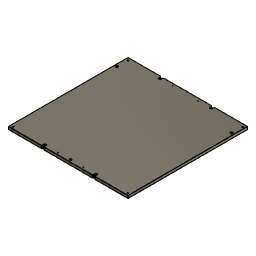
Voron_Universal_350x350_BuildPlate (Autodesk Fusion 360 design; units mm, degrees)
Autodesk Fusion 360 part; units mm, degrees
note: some values were not read from the file. Chosen so that the rebuilt part matches the saved one: how an offset face is resized; which pieces of a blend or face edit are solid.
sketch "Sketch1" plane through (0, 0, 0) normal (0, 1, 0) x (1, 0, 0)
  line L0 (0, 0) -> (351.6, 0)
  line L1 (351.6, 0) -> (351.6, 351.6)
  line L2 (351.6, 351.6) -> (0, 351.6)
  line L3 (0, 351.6) -> (0, 0)
  line L4 (175.8, 0) -> (100.8, 0)
  line L5 (100.8, 0) -> (100.8, 7)
  line L6 (100.8, 7) -> (175.8, 7) construction
  line L7 (175.8, 7) -> (175.8, 0) construction
  line L8 (351.6, 175.8) -> (300, 175.8) construction
  circle A0 centre (100.8, 7) radius 1.7
  circle A1 centre (250.8, 7) radius 1.7
  circle A2 centre (250.8, 344.6) radius 1.7
  circle A3 centre (100.8, 344.6) radius 1.7
  line L9 (0, 0) -> (7, 0)
  line L10 (7, 0) -> (7, 7) construction
  line L11 (7, 7) -> (0, 7) construction
  line L12 (0, 7) -> (0, 0)
  line L13 (351.6, 0) -> (344.6, 0)
  line L14 (344.6, 0) -> (344.6, 7) construction
  line L15 (344.6, 7) -> (351.6, 7) construction
  line L16 (351.6, 7) -> (351.6, 0)
  circle A4 centre (344.6, 7) radius 2.1
  circle A5 centre (7, 7) radius 2.1
  point P0 (250.8, 7)
  dimension "d1" = 351.6
  dimension "d2" = 351.6
  dimension "d3" = 75
  dimension "d4" = 7
  dimension "d5" = 3.4
  dimension "d6" = 7
  dimension "d7" = 7
  dimension "d8" = 7
  dimension "d9" = 7
  dimension "d10" = 4.2
  dimension "d11" = 4.2
  constraint horizontal L0
  constraint vertical L1
  constraint horizontal L2
  constraint vertical L3
  constraint coincident L0.start L3.end
  constraint horizontal L4
  constraint vertical L5
  constraint horizontal L6
  constraint vertical L7
  constraint midpoint L0 L4.start
  constraint midpoint L1 L8.start
  constraint perpendicular L1 L8
  constraint coincident L5.end L6.start
  constraint symmetric L7 L5.end P0
  constraint symmetric L7 A0 A1
  constraint symmetric L8 A0 A3
  constraint symmetric L8 A1 A2
  constraint horizontal L9
  constraint vertical L10
  constraint horizontal L11
  constraint vertical L12
  constraint horizontal L13
  constraint vertical L14
  constraint horizontal L15
  constraint vertical L16
  constraint coincident L14.end L15.start
  constraint coincident L10.end L11.start
  measures "d1" distance of L0.start L0.end
  measures "d2" distance of L0.start L2.end
  measures "d3" distance of L4.start L4.end
  measures "d4" distance of L4.start L6.end
  measures "d5" diameter of A0
  measures "d6" distance of L0.start L9.end
  measures "d7" distance of L0.start L11.end
  measures "d8" distance of L0.end L13.end
  measures "d9" distance of L0.end L15.end
  measures "d10" diameter of A4
  measures "d11" diameter of A5
extrude "Extrude1" add sketch "Sketch1" along normal blind 8 makes body 1
sketch "Sketch2" plane through (0, 8, 0) normal (0, 1, 0) x (-1, 0, 0)
  circle A0 centre (-250.8, -7) radius 1.7
  circle A1 centre (-250.8, -344.6) radius 1.7
  circle A2 centre (-100.8, -7) radius 1.7
  circle A3 centre (-344.6, -7) radius 2.1
  circle A4 centre (-7, -7) radius 2.1
  circle A5 centre (-100.8, -344.6) radius 1.7
  line L0 (-351.6, -351.6) -> (0, -351.6)
  line L1 (0, -351.6) -> (0, 0)
  line L2 (0, 0) -> (-351.6, 0)
  line L3 (-351.6, 0) -> (-351.6, -351.6)
  circle A6 centre (-100.8, -344.6) radius 3.25
  circle A7 centre (-250.8, -344.6) radius 3.25
  circle A8 centre (-100.8, -7) radius 3.25
  circle A9 centre (-250.8, -7) radius 3.25
  dimension "d14" = 6.5
  dimension "d15" = 6.5
  dimension "d16" = 6.5
  dimension "d17" = 6.5
  constraint concentric A5 A6
  constraint concentric A1 A7
  constraint concentric A2 A8
  constraint concentric A0 A9
  measures "d14" diameter of A6
  measures "d15" diameter of A7
  measures "d16" diameter of A8
  measures "d17" diameter of A9
extrude "Extrude2" cut sketch "Sketch2" against normal blind 3.5 contours A6 | A7 | A8 | A9 bodies 1
delete_face "DeleteFace1" 1 faces at (345.4637, 5.3333, -8.9142) on bodies 1
delete_face "DeleteFace2" 1 faces at (9.0974, 5.3333, -6.8953) on bodies 1
extrude "Extrude3" cut sketch "Sketch1" along normal blind 6 contours A4 | A5 bodies 1
thread "Thread1" "ISO Metric profile 5.0 M5x0.8 6H" major diameter 5.12 minor diameter 4.234 pitch 0.8 angle 60 resizes the face on face at (9.0974, 4, -6.8953) on face at (345.4637, 4, -8.9142) on bodies 1
copy_body "Body->Comp1" bodies 1 removing the originals makes body 2 in component "Component"
chamfer "Chamfer1" distance 0.2 angle 45 8 edges at (0, 0, -175.8) (175.8, 0, 0) (0, 8, -175.8) (175.8, 8, -351.6) (175.8, 0, -351.6) (351.6, 0, -175.8) (351.6, 8, -175.8) (175.8, 8, 0) on bodies 2 in component "Component"
fillet "Fillet1" radius 0.2 4 edges at (351.6, 4, 0) (0, 4, 0) (351.6, 4, -351.6) (0, 4, -351.6) on bodies 2 in component "Component"
delete_face "DeleteFace1'" 8 faces at (117.2667, 7.9333, -0.1333) (351.4667, 7.9333, -117.2667) (117.2667, 7.8667, -351.5333) (0.0667, 7.8667, -117.2667) (0.1333, 0.0667, -234.3333) (117.2667, 0.1333, -351.5333) (234.3333, 0.1333, -0.0667) (351.4667, 0.0667, -117.2667) on bodies 2 in component "Component"
sketch "Sketch3" plane through (0, 8, 0) normal (0, 1, 0) x (-1, 0, 0)
  line L0 (0, -351.4) -> (0, -0.2)
  arc A0 (0, -0.2) -> (-0.2, 0) centre (-0.2, -0.2) ccw
  line L1 (-0.2, 0) -> (-351.4, 0)
  arc A1 (-351.4, 0) -> (-351.6, -0.2) centre (-351.4, -0.2) ccw
  line L2 (-351.6, -0.2) -> (-351.6, -351.4)
  arc A2 (-351.6, -351.4) -> (-351.4, -351.6) centre (-351.4, -351.4) ccw
  line L3 (-351.4, -351.6) -> (-0.2, -351.6)
  arc A3 (-0.2, -351.6) -> (0, -351.4) centre (-0.2, -351.4) ccw
  circle A4 centre (-250.8, -344.6) radius 3.25
  circle A5 centre (-250.8, -7) radius 3.25
  circle A6 centre (-100.8, -344.6) radius 3.25
  circle A7 centre (-100.8, -7) radius 3.25
  line L4 (-250.8, -7) -> (-254.05, -7) construction
  line L5 (-250.8, -7) -> (-247.55, -7) construction
  line L6 (-254.05, -7) -> (-254.05, 0)
  line L7 (-247.55, -7) -> (-247.55, 0)
  constraint coincident A5.centre L4.start
  constraint coincident A5 L4.end
  constraint horizontal L4
  constraint coincident A5 L5.end
  constraint parallel L4 L5
  constraint coincident L1 L6.end
  constraint tangent A5 L6
  constraint coincident L1 L7.end
  constraint tangent A5 L7
extrude "Extrude1'" cut sketch "Sketch3" against normal blind 3.5 contours L1 A5 L6 L7 bodies 2 in component "Component"
sketch "Sketch4" plane through (0, 4.5, 0) normal (0, 1, 0) x (-1, 0, 0)
  circle A0 centre (-250.8, -7) radius 1.7
  arc A1 (-254.05, -7) -> (-247.55, -7) centre (-250.8, -7) ccw
  line L0 (-247.55, -7) -> (-247.55, 0)
  line L1 (-247.55, 0) -> (-254.05, 0)
  line L2 (-254.05, 0) -> (-254.05, -7)
  line L3 (-250.8, -7) -> (-252.5, -7) construction
  line L4 (-250.8, -7) -> (-249.1, -7) construction
  line L5 (-252.5, -7) -> (-252.5, 0)
  line L6 (-249.1, -7) -> (-249.1, 0)
  constraint coincident A0.centre A1.centre
  constraint coincident A0 L3.end
  constraint horizontal L3
  constraint coincident A0 L4.end
  constraint parallel L1 L4
  constraint coincident L1 L5.end
  constraint tangent A0 L5
  constraint coincident L1 L6.end
  constraint tangent A0 L6
extrude "Extrude2'" cut sketch "Sketch4" against normal blind 14 contours A0 L1 L5 L6 bodies 2 in component "Component"
fillet "Fillet2" radius 2 4 edges at (247.55, 6.25, 0) (249.1, 2.25, 0) (252.5, 2.25, 0) (254.05, 6.25, 0) on bodies 2 in component "Component"
ref_plane "WorkPlane1" through (175.8, 4, -175.8) normal (-1, 0, 0) x (0, 0, 1)
ref_plane "WorkPlane2" through (123.65, 4, -175.8) normal (0, 0, 1) x (1, 0, 0)
mirror "Mirror1" about plane through (175.8, 4, -175.8) normal (-1, 0, 0) of 11 faces at (246.0215, 5.6667, -0.0564) (247.55, 6.8333, -5.3333) (252.1367, 5.6667, -9.9624) (248.5833, 4.5, -3.6667) (247.4785, 1.5, -0.0361) (249.1, 3, -5.3333) (249.1084, 1.5, -7.1693) (252.5, 3, -5.3333) (254.0285, 1.5, -0.0564) (255.5785, 6.8333, -0.0564) (254.05, 6.8333, -5.3333) on bodies 2 in component "Component"
mirror "Mirror2" about plane through (123.65, 4, -175.8) normal (0, 0, 1) of 22 faces at (254.0285, 1.5, -0.0564) (255.5785, 6.8333, -0.0564) (254.05, 6.8333, -5.3333) (97.554, 5.6667, -7.162) (248.5833, 4.5, -3.6667) (252.5, 3, -5.3333) (102.4979, 1.5, -7.0847) (249.1, 3, -5.3333) (247.4785, 1.5, -0.0361) (246.0215, 5.6667, -0.0564) (247.55, 6.8333, -5.3333) (98.5475, 1.5, -0.6198) (99.1, 3, -5.3333) (249.1084, 1.5, -7.1693) (103.0167, 4.5, -3.6667) (252.1367, 5.6667, -9.9624) (97.55, 6.8333, -5.3333) (96.9302, 5.6667, -0.5525) (103.0525, 1.5, -0.6198) (104.6025, 5.6667, -0.6198) (104.05, 6.8333, -5.3333) (102.5, 3, -5.3333) on bodies 2 in component "Component"
chamfer "Chamfer4" distance 0.2 angle 45 64 edges at (0, 8, -175.8) (0.0586, 8, -0.0586) (47.875, 8, 0) (96.9642, 8, -0.5858) (97.55, 8, -4.5) (100.8, 8, -10.25) (104.05, 8, -4.5) (104.6358, 8, -0.5858) (175.8, 8, 0) (246.9642, 8, -0.5858) (247.55, 8, -4.5) (250.8, 8, -10.25) (254.05, 8, -4.5) (254.6358, 8, -0.5858) (303.725, 8, 0) (351.5414, 8, -0.0586) (351.6, 8, -175.8) (351.5414, 8, -351.5414) (303.725, 8, -351.6) (254.6358, 8, -351.0142) (254.05, 8, -347.1) (250.8, 8, -341.35) (247.55, 8, -347.1) (246.9642, 8, -351.0142) (175.8, 8, -351.6) (104.6358, 8, -351.0142) (104.05, 8, -347.1) (100.8, 8, -341.35) (97.55, 8, -347.1) (96.9642, 8, -351.0142) (47.875, 8, -351.6) (0.0586, 8, -351.5414) (48.65, 0, 0) (98.5142, 0, -0.5858) (99.1, 0, -4.5) (100.8, 0, -8.7) (102.5, 0, -4.5) (103.0858, 0, -0.5858) (175.8, 0, 0) (248.5142, 0, -0.5858) (249.1, 0, -4.5) (250.8, 0, -8.7) (252.5, 0, -4.5) (253.0858, 0, -0.5858) (302.95, 0, 0) (351.5414, 0, -0.0586) (351.6, 0, -175.8) (351.5414, 0, -351.5414) (302.95, 0, -351.6) (253.0858, 0, -351.0142) (252.5, 0, -347.1) (250.8, 0, -342.9) (249.1, 0, -347.1) (248.5142, 0, -351.0142) (175.8, 0, -351.6) (103.0858, 0, -351.0142) (102.5, 0, -347.1) (100.8, 0, -342.9) (99.1, 0, -347.1) (98.5142, 0, -351.0142) (48.65, 0, -351.6) (0.0586, 0, -351.5414) (0, 0, -175.8) (0.0586, 0, -0.0586) on bodies 2 in component "Component"
sketch "Sketch5" plane through (0, 8, 0) normal (0, 1, 0) x (-1, 0, 0)
  line L0 (-0.2, -0.2) -> (-95.55, -0.2)
  arc A0 (-95.55, -0.2) -> (-97.35, -2) centre (-95.55, -2) ccw
  line L1 (-97.35, -2) -> (-97.35, -7)
  arc A1 (-104.25, -7) -> (-97.35, -7) centre (-100.8, -7) ccw
  line L2 (-104.25, -7) -> (-104.25, -2)
  arc A2 (-104.25, -2) -> (-106.05, -0.2) centre (-106.05, -2) ccw
  line L3 (-106.05, -0.2) -> (-245.55, -0.2)
  arc A3 (-245.55, -0.2) -> (-247.35, -2) centre (-245.55, -2) ccw
  line L4 (-247.35, -2) -> (-247.35, -7)
  arc A4 (-254.25, -7) -> (-247.35, -7) centre (-250.8, -7) ccw
  line L5 (-254.25, -7) -> (-254.25, -2)
  arc A5 (-254.25, -2) -> (-256.05, -0.2) centre (-256.05, -2) ccw
  line L6 (-256.05, -0.2) -> (-351.4, -0.2)
  line L7 (-351.4, -0.2) -> (-351.4, -351.4)
  line L8 (-351.4, -351.4) -> (-256.05, -351.4)
  arc A6 (-256.05, -351.4) -> (-254.25, -349.6) centre (-256.05, -349.6) ccw
  line L9 (-254.25, -349.6) -> (-254.25, -344.6)
  arc A7 (-247.35, -344.6) -> (-254.25, -344.6) centre (-250.8, -344.6) ccw
  line L10 (-247.35, -344.6) -> (-247.35, -349.6)
  arc A8 (-247.35, -349.6) -> (-245.55, -351.4) centre (-245.55, -349.6) ccw
  line L11 (-245.55, -351.4) -> (-106.05, -351.4)
  arc A9 (-106.05, -351.4) -> (-104.25, -349.6) centre (-106.05, -349.6) ccw
  line L12 (-104.25, -349.6) -> (-104.25, -344.6)
  arc A10 (-97.35, -344.6) -> (-104.25, -344.6) centre (-100.8, -344.6) ccw
  line L13 (-97.35, -344.6) -> (-97.35, -349.6)
  arc A11 (-97.35, -349.6) -> (-95.55, -351.4) centre (-95.55, -349.6) ccw
  line L14 (-95.55, -351.4) -> (-0.2, -351.4)
  line L15 (-0.2, -351.4) -> (-0.2, -0.2)
  line L16 (-106.05, 0) -> (-245.55, 0)
  line L17 (-351.6, -0.2) -> (-351.6, -351.4)
  line L18 (-175.8, 0) -> (-175.8, -7) construction
  circle A12 centre (-175.8, -7) radius 1.7
  circle A13 centre (-175.8, -7) radius 3.25
  line L19 (-175.8, -7) -> (-175.8, -312) construction
  line L20 (-175.8, -312) -> (-351.6, -312) construction
  line L21 (-351.6, -312) -> (-344.6, -312) construction
  circle A14 centre (-344.6, -312) radius 1.7
  circle A15 centre (-344.6, -312) radius 3.25
  circle A16 centre (-7, -312) radius 3.25
  circle A17 centre (-7, -312) radius 1.7
  dimension "d36" = 7
  dimension "d37" = 3.4
  dimension "d38" = 6.5
  dimension "d39" = 305
  dimension "d40" = 7
  dimension "d41" = 3.4
  dimension "d42" = 6.5
  constraint midpoint L16 L18.start
  constraint perpendicular L3 L18
  constraint coincident L18.end A12.centre
  constraint parallel L18 L19
  constraint coincident L17 L20.end
  constraint perpendicular L17 L20
  constraint perpendicular L7 L21
  constraint coincident L21.end A14.centre
  constraint concentric A14 A15
  constraint symmetric L19 A14 A17
  constraint symmetric L19 A15 A16
  measures "d36" distance of L18.start L18.end
  measures "d37" diameter of A12
  measures "d38" diameter of A13
  measures "d39" distance of L18.end L19.end
  measures "d40" distance of L20.end L21.end
  measures "d41" diameter of A14
  measures "d42" diameter of A15
extrude "Extrude3'" cut sketch "Sketch5" against normal blind 30 contours A12 | A14 | A17 bodies 2 in component "Component"
extrude "Extrude4" cut sketch "Sketch5" against normal blind 3.5 contours A13 | A15 | A16 bodies 2 in component "Component"
chamfer "Chamfer5" distance 0.2 angle 45 3 edges at (10.0301, 8, -310.8247) (347.6301, 8, -310.8247) (178.8301, 8, -5.8247) on bodies 2 in component "Component"
delete_face "DeleteFace2'" 1 faces at (345.8358, 4, -8.7189) on bodies 2 in component "Component"
delete_face "DeleteFace3" 1 faces at (9.1144, 2, -7.1055) on bodies 2 in component "Component"
extrude "Extrude5" cut sketch "Sketch1" along normal blind 7 contours A4 | A5 bodies 2 in component "Component"
mirror "Mirror3" about plane through (123.65, 4, -175.8) normal (0, 0, 1) of "Extrude5" in component "Component"
sketch "Sketch6" plane through (0, 0, 0) normal (0, -1, 0) x (1, 0, 0)
  circle A0 centre (7, -344.6) radius 2.1
  circle A1 centre (344.6, -344.6) radius 2.1
  circle A2 centre (344.6, -7) radius 2.1
  circle A3 centre (7, -7) radius 2.1
  circle A4 centre (175.8, -7) radius 1.7
  circle A5 centre (344.6, -312) radius 1.7
  circle A6 centre (7, -312) radius 1.7
  line L0 (97.1, -0.2) -> (0.2, -0.2)
  line L1 (0.2, -0.2) -> (0.2, -351.4)
  line L2 (0.2, -351.4) -> (97.1, -351.4)
  arc A7 (97.1, -351.4) -> (98.9, -349.6) centre (97.1, -349.6) ccw
  line L3 (98.9, -349.6) -> (98.9, -344.6)
  arc A8 (102.7, -344.6) -> (98.9, -344.6) centre (100.8, -344.6) ccw
  line L4 (102.7, -344.6) -> (102.7, -349.6)
  arc A9 (102.7, -349.6) -> (104.5, -351.4) centre (104.5, -349.6) ccw
  line L5 (104.5, -351.4) -> (247.1, -351.4)
  arc A10 (247.1, -351.4) -> (248.9, -349.6) centre (247.1, -349.6) ccw
  line L6 (248.9, -349.6) -> (248.9, -344.6)
  arc A11 (252.7, -344.6) -> (248.9, -344.6) centre (250.8, -344.6) ccw
  line L7 (252.7, -344.6) -> (252.7, -349.6)
  arc A12 (252.7, -349.6) -> (254.5, -351.4) centre (254.5, -349.6) ccw
  line L8 (254.5, -351.4) -> (351.4, -351.4)
  line L9 (351.4, -351.4) -> (351.4, -0.2)
  line L10 (351.4, -0.2) -> (254.5, -0.2)
  arc A13 (254.5, -0.2) -> (252.7, -2) centre (254.5, -2) ccw
  line L11 (252.7, -2) -> (252.7, -7)
  arc A14 (248.9, -7) -> (252.7, -7) centre (250.8, -7) ccw
  line L12 (248.9, -7) -> (248.9, -2)
  arc A15 (248.9, -2) -> (247.1, -0.2) centre (247.1, -2) ccw
  line L13 (247.1, -0.2) -> (104.5, -0.2)
  arc A16 (104.5, -0.2) -> (102.7, -2) centre (104.5, -2) ccw
  line L14 (102.7, -2) -> (102.7, -7)
  arc A17 (98.9, -7) -> (102.7, -7) centre (100.8, -7) ccw
  line L15 (98.9, -7) -> (98.9, -2)
  arc A18 (98.9, -2) -> (97.1, -0.2) centre (97.1, -2) ccw
  line L16 (247.1, 0) -> (104.5, 0)
  line L17 (104.5, -351.6) -> (247.1, -351.6)
  line L18 (175.8, -351.6) -> (175.8, 0) construction
  line L19 (175.8, -175.8) -> (291.4366, -175.8) construction
  line L20 (175.8, -351.6) -> (175.8, -344.6) construction
  line L21 (175.8, -344.6) -> (138.3, -344.6) construction
  circle A19 centre (138.3, -344.6) radius 1.25
  circle A20 centre (213.3, -344.6) radius 1.25
  circle A21 centre (138.3, -7) radius 1.25
  circle A22 centre (213.3, -7) radius 1.25
  dimension "d52" = 7
  dimension "d53" = 37.5
  dimension "d54" = 2.5
  constraint midpoint L17 L18.start
  constraint midpoint L16 L18.end
  constraint midpoint L18 L19.start
  constraint perpendicular L18 L19
  constraint perpendicular L5 L20
  constraint perpendicular L18 L21
  constraint coincident L21.end A19.centre
  constraint symmetric L18 A19 A20
  constraint symmetric L19 A19 A21
  constraint symmetric L19 A20 A22
  measures "d52" distance of L18.start L20.end
  measures "d53" distance of L20.end L21.end
  measures "d54" diameter of A19
extrude "Extrude6" cut sketch "Sketch6" against normal blind 7 contours A19 | A20 | A21 | A22 bodies 2 in component "Component"
chamfer "Chamfer2" [suppressed] in component "Component"
chamfer "Chamfer3" [suppressed] in component "Component"
component "Component" placed x (1, 0, 0) y (0, 1, 0) z (0, 0, 1) at (0, 0, 0)
equation "d53 = ( 75 / 2 ) * 1 mm"
